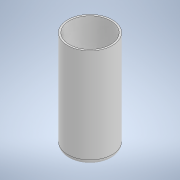
# Autodesk Inventor part: Exterior
Saved by Autodesk Inventor 2020 (Build 240168000, 168)
## iProperties
Created: 2020-10-28
Part Number: Exterior
Material: Generic
Document SubType Name: Modeling
Designer: aaron
Density: 1 g/cm^3
Appearance: Default
Author: aaron
Autodesk Inventor part; units mm, degrees
ref_plane "YZ Plane" through (0, 0, 0) normal (1, 0, 0) x (0, 1, 0)
ref_plane "XZ Plane" through (0, 0, 0) normal (0, 1, 0) x (-1, 0, 0)
ref_plane "XY Plane" through (0, 0, 0) normal (0, 0, 1) x (1, 0, 0)
sketch "Sketch1" plane through (0, 0, 0) normal (0, 0, 1) x (1, 0, 0)
  line L0 (0, 0) -> (35, 0)
  line L1 (45, 10) -> (45, 200)
  line L2 (0, 200) -> (0, 0)
  arc A0 (35, 0) -> (45, 10) centre (35, 10) ccw
  line L3 (41.5, 200) -> (41.5, 10)
  arc A1 (35, 3.5) -> (41.5, 10) centre (35, 10) ccw
  line L4 (35, 3.5) -> (0, 3.5)
  line L5 (41.5, 200) -> (45, 200)
  line L6 (0, 3.5) -> (0, 0)
  point P0 (45, 0)
  dimension "d0" = 90
  dimension "d1" = 200
  dimension "d2" = 10
  dimension "d5" = 3.5
  dimension "d6" = 3.5
  constraints: 14 end point, 4 point on circle, 3 point on line, 2 centre point, 2 horizontal, 2 perpendicular, 2 tangent, 2 vertical, 1 other
  measures "d0" diameter of L1 L2
  measures "d1" distance of point (45, 0) L1.end
  measures "d2" radius of A0
  measures "d5" distance between parallel lines of L0 L4
  measures "d6" distance between parallel lines of L1 L3
revolve "Revolution1" add sketch "Sketch1" angle 360 about axis through (0, 200, 0) along (0, -1, 0)
body "Solid1"
